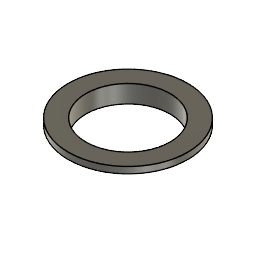
hx35_comp_outlet_ref (Autodesk Fusion 360 design; units mm, degrees)
part number: 2026-09-02-20-41-26-961
Autodesk Fusion 360 part; units mm, degrees
sketch "Sketch1" plane through (0, 0, 0) normal (0, 0, 1) x (1, 0, 0)
  circle A0 centre (0, 0) radius 26
  circle A1 centre (0, 0) radius 37
  circle A2 centre (0, 0) radius 27
  dimension "d3" = 52
  dimension "d4" = 74
  dimension "d7" = 1
  constraint coincident A0.centre A1.centre
  constraint concentric A0 A1
  measures "d3" diameter of A0
  measures "d4" diameter of A1
extrude "Extrude2" add sketch "Sketch1" along normal blind -7 and the other way blind -4 contours A2
extrude "Extrude3" add sketch "Sketch1" along normal blind 4 contours A1
equation "comp_outlet_bore = 52 mm"
equation "comp_outlet_OD = 74 mm"
equation "d3 = comp_outlet_bore"
equation "d4 = comp_outlet_OD"
